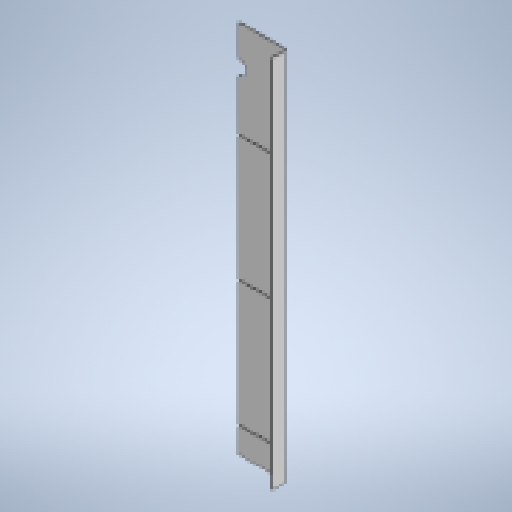
# Autodesk Inventor part: 0234 GBK stringer 1
Saved by Autodesk Inventor 2026.2 (Build 302298000, 298)
## iProperties
Created: 2026-05-07
Part Number: 0234 GBK stringer 1
Material: Steel
Document SubType Name: Sheet Metal
Designer: pokla
Density: 7.85 g/cm^3
Sheet Metal Rule: Default_mm
Appearance: Default
Author: admin
Autodesk Inventor part; units mm, degrees
ref_plane "YZ Plane" through (0, 0, 0) normal (1, 0, 0) x (0, 1, 0)
ref_plane "XZ Plane" through (0, 0, 0) normal (0, 1, 0) x (-1, 0, 0)
ref_plane "XY Plane" through (0, 0, 0) normal (0, 0, 1) x (1, 0, 0)
sketch "Sketch1" plane through (0, 0, 0) normal (0, 0, 1) x (1, 0, 0)
  line L0 (0, 1489) -> (-190.2469, 1489)
  line L1 (-190.2469, 1489) -> (-190.2469, 0)
  line L2 (-190.2469, 0) -> (0, 0)
  line L3 (0, 0) -> (0, 1489)
  line L4 (-190.2469, 100) -> (-66, 100)
  line L5 (-66, 100) -> (-66, 105)
  line L6 (-66, 105) -> (-190.2469, 105)
  line L7 (-190.2469, 105) -> (-190.2469, 100)
  line L8 (-190.2469, 600) -> (-66, 600)
  line L9 (-66, 600) -> (-66, 605)
  line L10 (-66, 605) -> (-190.2469, 605)
  line L11 (-190.2469, 605) -> (-190.2469, 600)
  line L12 (-190.2469, 1100) -> (-66, 1100)
  line L13 (-66, 1100) -> (-66, 1105)
  line L14 (-66, 1105) -> (-190.2469, 1105)
  line L15 (-190.2469, 1105) -> (-190.2469, 1100)
  circle A0 centre (-190.2469, 1335) radius 30
  point P0 (-190.2469, 605)
  point P1 (-190.2469, 1365)
  point P2 (-190.2469, 1305)
  dimension "d0" = 1489
  dimension "d1" = 190.2469
  dimension "d2" = 5
  dimension "d4" = 100
  dimension "d7" = 500
  dimension "d23" = 66
  dimension "d29" = 60
  dimension "d30" = 1335
  measures "d0" distance of L1.end L0.end
  measures "d1" distance of L1.end L2.end
  measures "d2" distance of L4.end L5.end
  measures "d4" distance between parallel lines of L2 L4
  measures "d7" distance of L4.start L8.start
  measures "d23" distance between parallel lines of L3 L5
  measures "d29" diameter of A0
  measures "d30" distance from line of A0.centre L2
extrude "Plate1" add sketch "Sketch1" along normal blind 4 contours L3 L2 L1 L4 L5 L6 L8 L9 L10 L12 L13 L14 A0 L0
sketch "Sketch2" plane through (-4, 1489, 0) normal (1, 0, 0) x (0, 1, 0)
  line L0 (-1489, 0) -> (0, 0)
  line L1 (0, 0) -> (0, 60)
  line L2 (0, 60) -> (-1489, 60)
  line L3 (-1489, 60) -> (-1489, 0)
  constraints: 6 end point, 1 horizontal, 1 perpendicular, 1 vertical
edge flange "Flange1" height 60 angle 90 thickness 4 bend radius 4 thickness toward (1, 0, 0) relief straight relief width 4 relief depth 2 edges at (0, 744.5, 4) wall of the first edge with corners at (-4, 0, 0) (-4, 1489, 0) (-4, 1489, 60) (-4, 0, 60)
bend "Bend1"
corner "Corner1"
chamfer "Corner Chamfer1" distance 3 angle 45 6 edges at (-190.2469, 100, 2) (-190.2469, 105, 2) (-190.2469, 600, 2) (-190.2469, 605, 2) (-190.2469, 1105, 2) (-190.2469, 1100, 2)
equation "\"d0\" = Стрингер_длина"
equation "\"d1\" = стрингер_глубина_1"
equation "\"d2\" = паз_под_стрингер_толщина"
equation "\"d23\" = паз_под_стрингер_глубина - Thickness"
equation "\"d29\" = 2 * радиус_выреза_под_сварку"
equation "\"d12\" = Thickness"
equation "\"d13\" = BendReliefWidth"
equation "\"d14\" = BendReliefDepth"
equation "\"d15\" = MinimumRemnant"
equation "\"d16\" = TransitionRadius"
equation "\"d17\" = ребро_усилителей"
equation "\"d19\" = BendRadius"
equation "\"d20\" = CornerReliefSize"
equation "\"d21\" = GapSize"
equation "\"d22\" = JacobiRadiusSize"
equation "\"BendRadius\" = Thickness"
equation "\"BendReliefWidth\" = Thickness"
equation "\"BendReliefDepth\" = 0.5 * Thickness"
equation "\"CornerReliefSize\" = 4 * Thickness"
equation "\"MinimumRemnant\" = 2 * Thickness"
equation "\"TransitionRadius\" = BendRadius"
equation "\"JacobiRadiusSize\" = BendRadius"
equation "\"GapSize\" = Thickness"
equation "\"Стрингер_длина\" = 1489"
equation "\"стрингер_глубина_1\" = 190.246925"
equation "\"паз_под_стрингер_толщина\" = 5"
equation "\"паз_под_стрингер_глубина\" = 70"
equation "\"Thickness\" = 4"
equation "\"радиус_выреза_под_сварку\" = 30"
equation "\"ребро_усилителей\" = 60"
body "Solid1"
